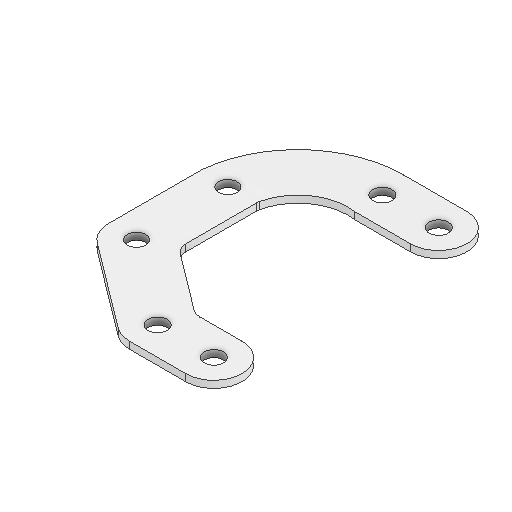
# Autodesk Inventor part: Rear Gusset
Saved by Autodesk Inventor 2025 (Build 290162000, 162)
## iProperties
Created: 2025-02-12
Part Number: Rear Gusset
Material: Acetal Resin, White
Document SubType Name: Modeling
Designer: Averey Ku
Density: 1.425 g/cm^3
Appearance: Smooth - White
Author: Averey Ku
Autodesk Inventor part; units mm, degrees
ref_plane "YZ Plane" through (0, 0, 0) normal (1, 0, 0) x (0, 1, 0)
ref_plane "XZ Plane" through (0, 0, 0) normal (0, 1, 0) x (-1, 0, 0)
ref_plane "XY Plane" through (0, 0, 0) normal (0, 0, 1) x (1, 0, 0)
sketch "gusset" plane through (0, 0, 0) normal (0, 0, 1) x (1, 0, 0)
  circle A0 centre (-8.9225, 14.8571) radius 2.1844
  circle A1 centre (-21.6225, 14.8571) radius 2.1844
  arc A2 (-21.6225, 21.2071) -> (-21.6225, 8.5071) centre (-21.6225, 14.8571) ccw
  arc A3 (-5.1125, 19.9371) -> (-8.9225, 21.2071) centre (-8.9225, 14.8571) ccw
  line L0 (16.4775, 0.5696) -> (16.4775, -20.0679)
  line L1 (3.7775, -20.1515) -> (3.7775, -4.1929)
  line L2 (2.5075, -1.6529) -> (-10.1925, 7.8721)
  line L3 (-21.6225, 8.5071) -> (-12.0975, 8.5071)
  line L4 (-21.6225, 21.2071) -> (-8.9225, 21.2071)
  arc A4 (16.4775, 0.5696) -> (13.9375, 5.6496) centre (10.1275, 0.5696) ccw
  line L5 (-5.1125, 19.9371) -> (13.9375, 5.6496)
  circle A5 centre (-21.6232, -35.9429) radius 2.1844
  circle A6 centre (-8.9225, -35.9429) radius 2.1844
  line L6 (-21.6246, -29.5943) -> (-8.9205, -29.5916)
  line L7 (-21.6233, -42.2916) -> (-7.3358, -42.2916)
  arc A7 (-21.6246, -29.5943) -> (-21.6233, -42.2916) centre (-21.6232, -35.9429) ccw
  circle A8 centre (10.1275, 0.5696) radius 2.0955
  circle A9 centre (10.1275, -20.0679) radius 2.0955
  arc A10 (3.7775, -4.1929) -> (2.5075, -1.6529) centre (0.6025, -4.1929) ccw
  arc A11 (-10.1925, 7.8721) -> (-12.0975, 8.5071) centre (-12.0975, 5.3321) ccw
  arc A12 (-7.3358, -42.2916) -> (16.4487, -20.6722) centre (-7.3358, -18.3986) ccw
  arc A13 (16.4487, -20.6722) -> (16.4775, -20.0679) centre (10.1275, -20.0679) ccw
  arc A14 (-8.9205, -29.5916) -> (3.7028, -20.8361) centre (-7.3358, -18.3986) ccw
  arc A15 (3.7028, -20.8361) -> (3.7775, -20.1515) centre (0.6025, -20.1515) ccw
  point P0 (-7.0147, -10.522)
  point P1 (16.4775, -20.3474)
  point P2 (3.7775, -20.4691)
  point P3 (4.4125, 12.7933)
  dimension "d0" = 12.7
  dimension "d2" = 12.7
  dimension "d3" = 4.191
  dimension "d4" = 3.175
  dimension "d8" = 12.7
  dimension "d12" = 14.2875
  dimension "d13" = 6.35
  dimension "d14" = 15.875
  dimension "d15" = 3.175
  measures "d0" diameter of A4
  measures "d3" diameter of A8
  measures "d4" radius of A10
  measures "d8" distance from line of L2 point (4.412, 12.793)
  measures "d12" distance of L7.start L7.end
  measures "d13" radius of A13
  measures "d14" vertical distance of A6.centre A9.centre
  measures "d15" radius of A15
sketch "Sketch1" plane through (0, 0, 0) normal (0, 1, 0) x (-1, 0, 0)
  circle A0 centre (12.7, 0) radius 2.1844
  circle A1 centre (0, 0) radius 2.1844
  arc A2 (0, 6.35) -> (0, -6.35) centre (0, 0) ccw
  arc A3 (16.51, 5.08) -> (12.7, 6.35) centre (12.7, 0) ccw
  line L0 (38.1, -14.2875) -> (38.1, -34.925)
  line L1 (25.4, -35.0086) -> (25.4, -19.05)
  line L2 (24.13, -16.51) -> (11.43, -6.985)
  line L3 (0, -6.35) -> (9.525, -6.35)
  line L4 (0, 6.35) -> (12.7, 6.35)
  arc A4 (38.1, -14.2875) -> (35.56, -9.2075) centre (31.75, -14.2875) ccw
  line L5 (16.51, 5.08) -> (35.56, -9.2075)
  circle A5 centre (-0.0007, -50.8) radius 2.1844
  circle A6 centre (12.7, -50.8) radius 2.1844
  line L6 (-0.0021, -44.4514) -> (12.702, -44.4486)
  line L7 (-0.0008, -57.1486) -> (14.2867, -57.1486)
  arc A7 (-0.0021, -44.4514) -> (-0.0008, -57.1486) centre (-0.0007, -50.8) ccw
  circle A8 centre (31.75, -14.2875) radius 2.0955
  circle A9 centre (31.75, -34.925) radius 2.0955
  arc A10 (25.4, -19.05) -> (24.13, -16.51) centre (22.225, -19.05) ccw
  arc A11 (11.43, -6.985) -> (9.525, -6.35) centre (9.525, -9.525) ccw
  arc A12 (14.2867, -57.1486) -> (38.0712, -35.5292) centre (14.2867, -33.2557) ccw
  arc A13 (38.0712, -35.5292) -> (38.1, -34.925) centre (31.75, -34.925) ccw
  arc A14 (12.702, -44.4486) -> (25.3253, -35.6931) centre (14.2867, -33.2557) ccw
  arc A15 (25.3253, -35.6931) -> (25.4, -35.0086) centre (22.225, -35.0086) ccw
  constraints: 1 other
extrude "Extrusion1" add sketch "Sketch1" along normal blind 1.5875
body "Solid1"
